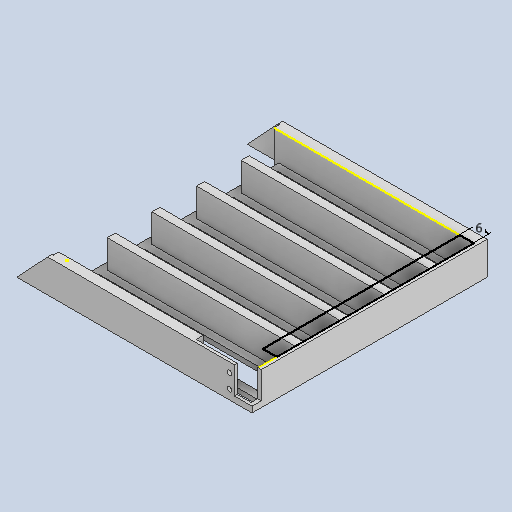
# Autodesk Inventor part: Case
Saved by Autodesk Inventor 2023 (Build 270158000, 158)
## iProperties
Created: 2024-03-21
Part Number: Case
Material: Generic
Document SubType Name: Modeling
Designer: noname
Density: 1 g/cm^3
Appearance: Default
Author: noname
Autodesk Inventor part; units mm, degrees
ref_plane "YZ Plane" through (0, 0, 0) normal (1, 0, 0) x (0, 1, 0)
ref_plane "XZ Plane" through (0, 0, 0) normal (0, 1, 0) x (-1, 0, 0)
ref_plane "XY Plane" through (0, 0, 0) normal (0, 0, 1) x (1, 0, 0)
sketch "Sketch1" plane through (0, 0, 0) normal (1, 0, 0) x (0, 1, 0)
  line L0 (0, 5) -> (0, -5)
  line L1 (0, -5) -> (2, -5)
  line L2 (2, -5) -> (2, -1.7)
  line L3 (2, -1.7) -> (14, -1.7)
  line L4 (14, -1.7) -> (14, 1.7)
  line L5 (0, 0) -> (14, 0)
  line L6 (0, 5) -> (2, 5)
  line L7 (2, 5) -> (2, 1.7)
  line L8 (2, 1.7) -> (14, 1.7)
  dimension "d0" = 3.4
  dimension "d1" = 10
  dimension "d2" = 2
  dimension "d3" = 14
  constraints: 18 end point, 2 horizontal, 2 midpoint, 2 perpendicular, 2 symmetric about line, 2 vertical, 1 coincident
  measures "d0" distance between parallel lines of L3 L8
  measures "d1" distance between parallel lines of L1 L6
  measures "d2" distance between parallel lines of L0 L7
  measures "d3" distance between parallel lines of L0 L4
extrude "Extrusion1" add sketch "Sketch1" along normal blind 76
pattern_linear "Rectangular Pattern1" count 6 spacing 19 along (0, 0, -1) of "Extrusion1"
sketch "Sketch3" plane through (76, 0, 0) normal (1, 0, 0) x (0, 0, -1)
  line L0 (-1.7, 2) -> (-5, 2) projected
  line L1 (-1.7, 2) -> (-5, 2)
  line L2 (-5, 2) -> (-5, 14)
  line L3 (-5, 14) -> (-1.7, 14)
  line L4 (-1.7, 14) -> (-1.7, 2)
  line L5 (96.7, 2) -> (96.7, 14) projected
  line L6 (96.7, 2) -> (100, 2)
  line L7 (100, 2) -> (100, 14)
  line L8 (100, 14) -> (96.7, 14)
  line L9 (96.7, 14) -> (96.7, 2)
  point P0 (0, 0)
  constraints: 16 end point, 4 parallel, 3 coincident, 2 horizontal, 2 perpendicular, 1 point on line
extrude "Extrusion2" add sketch "Sketch3" against normal up to surface (76 mm away)
sketch "Sketch4" plane through (76, 0, 0) normal (1, 0, 0) x (0, 0, -1)
  line L0 (1.7, 14) -> (-5, 14) projected
  line L1 (90, 0) -> (100, 0) projected
  line L2 (-2.5, 14) -> (97.5, 14)
  line L3 (97.5, 14) -> (97.5, 0)
  line L4 (97.5, 0) -> (-2.5, 0)
  line L5 (-2.5, 0) -> (-2.5, 14)
  line L6 (43, 0) -> (43, 2) projected
  line L7 (55.3, 2) -> (52, 2) projected
  line L8 (43, 2) -> (52, 2)
  point P0 (0, 0)
  point P1 (47.5, 2)
  point P2 (47.5, 0)
  dimension "d12" = 100
  constraints: 10 end point, 2 horizontal, 2 midpoint, 2 parallel, 2 point on line, 1 perpendicular, 1 vertical alignment
  measures "d12" distance between parallel lines of L3 L5
extrude "Extrusion3" cut sketch "Sketch4" against normal through all keep common part
sketch "Sketch5" plane through (76, 0, 0) normal (1, 0, 0) x (0, 0, -1)
  line L0 (-2.5, 0) -> (5, 0) projected
  line L1 (97.5, 14) -> (97.5, 0) projected
  line L2 (-2.5, 0) -> (97.5, 0)
  line L3 (97.5, 0) -> (97.5, 2)
  line L4 (97.5, 2) -> (-2.5, 2)
  line L5 (-2.5, 2) -> (-2.5, 0)
  point P0 (0, 0)
  point P1 (90, 2)
  point P2 (97.5, 0)
  constraints: 8 end point, 2 parallel, 2 point on line, 1 horizontal, 1 perpendicular
extrude "Extrusion4" add sketch "Sketch5" along normal blind 5.4
sketch "Sketch7" plane through (0, 2, -1.7) normal (0, 1, 0) x (1, 0, 0)
  line L0 (76, -4.2) -> (76, 0) projected
  line L1 (76, 0) -> (79.8, 0)
  line L2 (79.8, 0) -> (79.8, 91.6)
  line L3 (79.8, 91.6) -> (76, 91.6)
  line L4 (76, 0) -> (76, -4.2) projected
  line L5 (81.4, 95.8) -> (81.4, -4.2) projected
  line L6 (0, 3.3) -> (0, 0) projected
  line L7 (0, 0) -> (76, 0) projected
  line L8 (76, -4.2) -> (76, 0) projected
  line L9 (76, -4.2) -> (81.4, -4.2) projected
  line L10 (81.4, 95.8) -> (81.4, -4.2) projected
  line L11 (76, 95.8) -> (81.4, 95.8) projected
  line L12 (76, 91.6) -> (76, 95.8) projected
  line L13 (0, 91.6) -> (76, 91.6) projected
  line L14 (0, 91.6) -> (0, 88.3) projected
  line L15 (0, 88.3) -> (76, 88.3) projected
  line L16 (76, 88.3) -> (76, 79.3) projected
  line L17 (0, 79.3) -> (76, 79.3) projected
  line L18 (0, 79.3) -> (0, 76) projected
  line L19 (0, 76) -> (76, 76) projected
  line L20 (76, 72.6) -> (76, 76) projected
  line L21 (0, 72.6) -> (76, 72.6) projected
  line L22 (0, 72.6) -> (0, 69.3) projected
  line L23 (0, 69.3) -> (76, 69.3) projected
  line L24 (76, 69.3) -> (76, 60.3) projected
  line L25 (0, 60.3) -> (76, 60.3) projected
  line L26 (0, 60.3) -> (0, 57) projected
  line L27 (0, 57) -> (76, 57) projected
  line L28 (76, 53.6) -> (76, 57) projected
  line L29 (0, 53.6) -> (76, 53.6) projected
  line L30 (0, 53.6) -> (0, 50.3) projected
  line L31 (0, 50.3) -> (76, 50.3) projected
  line L32 (76, 50.3) -> (76, 41.3) projected
  line L33 (0, 41.3) -> (76, 41.3) projected
  line L34 (0, 41.3) -> (0, 38) projected
  line L35 (0, 38) -> (76, 38) projected
  line L36 (76, 34.6) -> (76, 38) projected
  line L37 (0, 34.6) -> (76, 34.6) projected
  line L38 (0, 34.6) -> (0, 31.3) projected
  line L39 (0, 31.3) -> (76, 31.3) projected
  line L40 (76, 31.3) -> (76, 22.3) projected
  line L41 (0, 22.3) -> (76, 22.3) projected
  line L42 (0, 22.3) -> (0, 19) projected
  line L43 (0, 19) -> (76, 19) projected
  line L44 (76, 15.6) -> (76, 19) projected
  line L45 (0, 15.6) -> (76, 15.6) projected
  line L46 (0, 15.6) -> (0, 12.3) projected
  line L47 (0, 12.3) -> (76, 12.3) projected
  line L48 (76, 12.3) -> (76, 3.3) projected
  line L49 (0, 3.3) -> (76, 3.3) projected
  point P0 (0, -1.7)
  point P1 (81.4, -4.2)
  dimension "d17" = 1.6
  constraints: 6 end point, 2 perpendicular, 1 coincident, 1 horizontal
  measures "d17" distance between parallel lines of L5 L2
extrude "Extrusion5" add sketch "Sketch7" along normal up to surface (12 mm away) contours L0 L1 L2 L3 L12 L11 L5 L9
sketch "Sketch8" plane through (76, 2, -58.7) normal (1, 0, 0) x (0, 0, -1)
  line L0 (-41.4, 0) -> (-38, 0) projected
  line L1 (-38, 0) -> (-38, 12) projected
  line L2 (-38, 12) -> (-41.4, 12) projected
  line L3 (-41.4, 12) -> (-41.4, 0) projected
  line L4 (-22.4, 0) -> (-19, 0) projected
  line L5 (-19, 0) -> (-19, 12) projected
  line L6 (-19, 12) -> (-22.4, 12) projected
  line L7 (-22.4, 12) -> (-22.4, 0) projected
  line L8 (-3.4, 0) -> (0, 0) projected
  line L9 (0, 0) -> (0, 12) projected
  line L10 (0, 12) -> (-3.4, 12) projected
  line L11 (-3.4, 12) -> (-3.4, 0) projected
  line L12 (15.6, 0) -> (19, 0) projected
  line L13 (19, 0) -> (19, 12) projected
  line L14 (19, 12) -> (15.6, 12) projected
  line L15 (15.6, 12) -> (15.6, 0) projected
  point P0 (-58.7, -2)
extrude "Extrusion6" add sketch "Sketch8" along normal through all
sketch "Sketch9" plane through (0, 2, -93.3) normal (-1, 0, 0) x (0, 0, 1)
  line L0 (-4.2, -2) -> (-4.2, 12) projected
  line L1 (95.8, -2) -> (95.8, 12) projected
  line L2 (-4.2, -2) -> (95.8, -2)
  line L3 (95.8, -2) -> (95.8, 0)
  line L4 (95.8, 0) -> (-4.2, 0)
  line L5 (-4.2, 0) -> (-4.2, -2)
  line L6 (-4.2, -2) -> (-4.2, 12) projected
  line L7 (3.3, -2) -> (-4.2, -2) projected
  line L8 (3.3, 0) -> (3.3, -2) projected
  line L9 (0, 0) -> (3.3, 0) projected
  line L10 (0, 12) -> (0, 0) projected
  line L11 (0, 12) -> (-4.2, 12) projected
  line L12 (95.8, 12) -> (95.8, -2) projected
  line L13 (91.6, 12) -> (95.8, 12) projected
  line L14 (91.6, 0) -> (91.6, 12) projected
  line L15 (88.3, 0) -> (91.6, 0) projected
  line L16 (88.3, -2) -> (88.3, 0) projected
  line L17 (95.8, -2) -> (88.3, -2) projected
  point P0 (93.3, -2)
  point P1 (95.8, 12)
  constraints: 8 end point, 2 parallel, 2 point on line, 1 horizontal, 1 perpendicular
extrude "Extrusion7" add sketch "Sketch9" along normal blind 5
chamfer "Chamfer1" distance 2 angle 45 1 edges at (-5, 2, -47.5)
sketch "Sketch11" plane through (81.4, 0, -97.5) normal (0, 0, -1) x (-1, 0, 0)
  line L0 (86.4, 0) -> (86.4, 14) projected
  line L1 (86.4, 0) -> (100, 0)
  line L2 (100, 0) -> (86.9767, 14)
  line L3 (86.4, 14) -> (1.6, 14) projected
  line L4 (0, 0) -> (0, 14) projected
  line L5 (86.4, 14) -> (0, 14) projected
  line L6 (0, 0) -> (0, 14) projected
  line L7 (0, 0) -> (86.4, 0) projected
  line L8 (86.4, 14) -> (86.4, 0) projected
  line L9 (86.9767, 14) -> (86.4, 14)
  point P0 (81.4, 0)
  point P1 (86.4, 7.12)
  point P2 (1.6, 14)
  dimension "d29" = 47.07
  dimension "d36" = 100
  constraints: 6 end point, 2 horizontal, 1 point on line
  measures "d29" angle of L1 L2
  measures "d36" distance from line of L4 L1.end
extrude "Extrusion8" add sketch "Sketch11" against normal blind 2 contours L0 L9 L2 L1
ref_plane "Work Plane1" through (81.4, 0, -47.5) normal (0, 0, -1) x (-1, 0, 0)
mirror "Mirror1" about plane through (81.4, 0, -47.5) normal (0, 0, -1) of "Extrusion8"
sketch "Sketch14" plane through (81.4, 14, 2.5) normal (0, 1, 0) x (1, 0, 0)
  line L0 (-86.4, 4.2) -> (-1.6, 4.2) projected
  line L1 (-1.6, 4.2) -> (-25, 4.2)
  line L2 (-25, 4.2) -> (-25, 1.2)
  line L3 (-25, 1.2) -> (-1.6, 1.2)
  line L4 (-1.6, 1.2) -> (-1.6, 4.2)
  point P0 (-81.4, 2.5)
  dimension "d37" = 3
  dimension "d38" = 23.4
  constraints: 8 end point, 2 parallel, 1 horizontal, 1 perpendicular
  measures "d37" distance between parallel lines of L0 L3
  measures "d38" distance between parallel lines of L4 L2
extrude "Extrusion11" cut sketch "Sketch14" against normal through all
sketch "Sketch15" plane through (81.4, 0, 2.5) normal (0, 0, 1) x (1, 0, 0)
  line L0 (0, 0) -> (0, 14) projected
  line L1 (0, 14) -> (-7.5, 14)
  line L2 (-7.5, 14) -> (-7.5, 2.5)
  line L3 (-7.5, 2.5) -> (0, 2.5)
  line L4 (0, 2.5) -> (0, 14)
  point P0 (-81.4, 0)
  point P1 (0, 2.5)
  dimension "d41" = 11.5
  dimension "d42" = 7.5
  constraints: 8 end point, 2 parallel, 1 horizontal, 1 perpendicular
  measures "d41" distance between parallel lines of L1 L3
  measures "d42" distance between parallel lines of L0 L2
extrude "Extrusion12" cut sketch "Sketch15" against normal blind 4
sketch "Sketch17" plane through (-18.6, 0, 2.5) normal (0, 0, 1) x (1, 0, 0)
  line L0 (100, 0) -> (0, 0) projected
  point P0 (18.6, 0)
  point P1 (90.4317, 10)
  point P2 (90.4317, 4)
  dimension "d52" = 6
  dimension "d53" = 4
  constraints: 1 vertical alignment
  measures "d52" distance of point (90.432, 4) point (90.432, 10)
  measures "d53" distance from line of L0 point (90.432, 4)
hole "Hole1" at (71.8317, 10, 2.5) at (71.8317, 4, 2.5) direction (0, 0, -1) diameter 2 depth 19.8
sketch "Sketch18" plane through (0, 14, -77.7) normal (0, 1, 0) x (1, 0, 0)
  line L0 (79.8, -76) -> (79.8, -60.4) projected
  line L1 (-5, 15.6) -> (79.8, 15.6) projected
  line L2 (79.8, -68.2) -> (73.8, -68.2)
  line L3 (73.8, -68.2) -> (73.8, 15.6)
  line L4 (73.8, 15.6) -> (79.8, 15.6)
  line L5 (79.8, 15.6) -> (79.8, -68.2)
  point P0 (0, -77.7)
  dimension "d54" = 6
  constraints: 8 end point, 2 parallel, 1 horizontal, 1 midpoint, 1 perpendicular, 1 point on line
  measures "d54" distance between parallel lines of L5 L3
body "Solid1"
